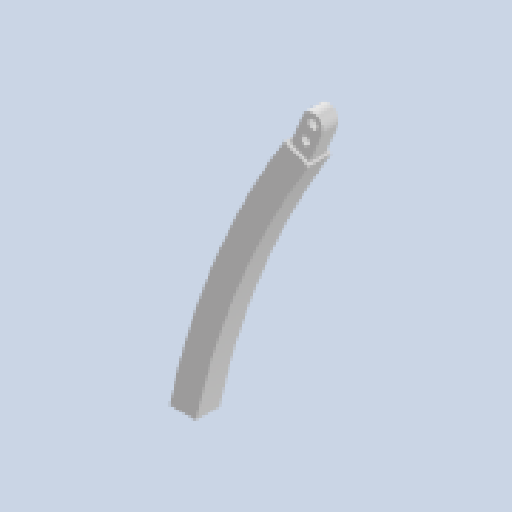
# Autodesk Inventor part: Picior
Saved by Autodesk Inventor 2025.2 (Build 292293000, 293)
## iProperties
Created: 2025-03-29
Part Number: Picior
Material: Generic
Document SubType Name: Modeling
Designer: mirewn
Density: 1 g/cm^3
Appearance: Default
Author: mirewn
Autodesk Inventor part; units mm, degrees
ref_plane "YZ Plane" through (0, 0, 0) normal (1, 0, 0) x (0, 1, 0)
ref_plane "XZ Plane" through (0, 0, 0) normal (0, 1, 0) x (-1, 0, 0)
ref_plane "XY Plane" through (0, 0, 0) normal (0, 0, 1) x (1, 0, 0)
sketch "Sketch1" plane through (0, 0, 0) normal (0, 0, 1) x (1, 0, 0)
  circle A0 centre (0, 0) radius 1.5
  arc A1 (20, -14.1391) -> (-59, 12.7093) centre (-111.8451, -272.4352) ccw
  line L0 (-111.8451, -272.4352) -> (0, 0) construction
  line L1 (0, 0) -> (4.5612, 11.1102) construction
  circle A2 centre (2.4686, 6.013) radius 1.5
  arc A3 (5.7063, 4.6838) -> (-0.7692, 7.3422) centre (2.4686, 6.013) ccw
  line L2 (5.7063, 4.6838) -> (1.5207, -5.5116)
  line L3 (-0.7692, 7.3422) -> (-4.9548, -2.8532)
  arc A4 (2.4871, -5.769) -> (-35.99, -100) centre (256.9615, -164.6487) ccw
  arc A5 (-5.885, -2.4862) -> (-45.041, -100) centre (256.9615, -164.6487) ccw
  line L4 (-35.99, -100) -> (-45.041, -100)
  arc A6 (2.5858, -6.2386) -> (-6.5507, -2.4942) centre (-111.8451, -272.4352) ccw
  line L5 (-4.9548, -2.8532) -> (-5.0498, -3.0844)
  line L6 (1.5207, -5.5116) -> (1.4258, -5.7429)
  point P0 (-40.5155, -100)
  point P1 (-4.9548, -2.8532)
  point P2 (2.4107, -5.8913)
  point P3 (2.2769, -6.106)
  point P4 (-6.0183, -2.7024)
  point P5 (-4.9548, -2.8532)
  dimension "d4" = 3
  dimension "d5" = 294.5
  dimension "d7" = 3
  dimension "d8" = 6.5
  dimension "d9" = 3.5
  dimension "d10" = 300
  dimension "d11" = 1
  dimension "d12" = 1
  dimension "d13" = 100
  dimension "d18" = 289.75
  constraints: 14 end point, 14 point on circle, 7 centre point, 3 coincident, 2 parallel, 2 point on line, 2 symmetric about line, 1 horizontal, 1 midpoint, 1 tangent, 2 other
  measures "d4" diameter of A0
  measures "d5" distance of L0.start L0.end
  measures "d7" diameter of A2
  measures "d8" distance of L0.end A2.centre
  measures "d9" radius of A3
  measures "d10" radius of A4
  measures "d11" distance of A4.start L2.end
  measures "d12" distance of L3.end A5.start
  measures "d13" vertical distance of L0.end point (-40.516, -100)
  measures "d18" radius of A6
extrude "Extrusion1" add sketch "Sketch1" along normal mid plane 5.5 contours L6 A6 L5 A1 | A1 L3 A3 L2
extrude "Extrusion2" add sketch "Sketch1" along normal mid plane 8 contours A6 A4 L4 A5
body "Solid1"
